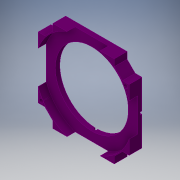
# Autodesk Inventor part: 20_Cube_Insert_CirAp_Lid
Saved by Autodesk Inventor 2019.4 (Build 234330000, 330)
## iProperties
Created: 2019-10-23
Part Number: 20_Cube_Insert_CirAp_Lid
Material: Generic
Document SubType Name: Modeling
Designer: marsikovabarbora
Density: 1 g/cm^3
Appearance: Default
Author: marsikovabarbora
Autodesk Inventor part; units mm, degrees
ref_plane "YZ Plane" through (0, 0, 0) normal (1, 0, 0) x (0, 1, 0)
ref_plane "XZ Plane" through (0, 0, 0) normal (0, 1, 0) x (-1, 0, 0)
ref_plane "XY Plane" through (0, 0, 0) normal (0, 0, 1) x (1, 0, 0)
sketch "Sketch1" plane through (0, 0, 0) normal (0, 0, 1) x (1, 0, 0)
  line L0 (-34.8609, 0) -> (34.8609, 0) construction
  line L1 (0, -34.8609) -> (0, 34.8609) construction
  line L2 (0, 0) -> (11.6542, 11.6542) construction
  line L3 (0, 0) -> (16.4815, 0) construction
  line L4 (0, 24.9006) -> (16.8, 24.9006)
  line L5 (16.8, 24.9006) -> (16.8, 21.2406)
  line L6 (16.8, 21.2406) -> (19.0203, 19.0203)
  line L7 (24.9006, 0) -> (24.9006, 16.8)
  line L8 (24.9006, 16.8) -> (21.2406, 16.8)
  line L9 (21.2406, 16.8) -> (19.0203, 19.0203)
  line L10 (0, 0) -> (-11.6542, 11.6542) construction
  line L11 (0, 0) -> (-16.4815, 0) construction
  line L12 (0, 24.9006) -> (-16.8, 24.9006)
  line L13 (-16.8, 24.9006) -> (-16.8, 21.2406)
  line L14 (-16.8, 21.2406) -> (-19.0203, 19.0203)
  line L15 (-24.9006, 0) -> (-24.9006, 16.8)
  line L16 (-24.9006, 16.8) -> (-21.2406, 16.8)
  line L17 (-21.2406, 16.8) -> (-19.0203, 19.0203)
  line L18 (0, 0) -> (11.6542, -11.6542) construction
  line L19 (0, -24.9006) -> (16.8, -24.9006)
  line L20 (16.8, -24.9006) -> (16.8, -21.2406)
  line L21 (16.8, -21.2406) -> (19.0203, -19.0203)
  line L22 (24.9006, 0) -> (24.9006, -16.8)
  line L23 (24.9006, -16.8) -> (21.2406, -16.8)
  line L24 (21.2406, -16.8) -> (19.0203, -19.0203)
  line L25 (0, 0) -> (-11.6542, -11.6542) construction
  line L26 (0, -24.9006) -> (-16.8, -24.9006)
  line L27 (-16.8, -24.9006) -> (-16.8, -21.2406)
  line L28 (-16.8, -21.2406) -> (-19.0203, -19.0203)
  line L29 (-24.9006, 0) -> (-24.9006, -16.8)
  line L30 (-24.9006, -16.8) -> (-21.2406, -16.8)
  line L31 (-21.2406, -16.8) -> (-19.0203, -19.0203)
  dimension "d0" = 45
  dimension "d1" = 3.14
  dimension "d2" = 3.66
  dimension "d3" = 16.8
  constraints: 60 end point, 24 symmetric about line, 5 point on line, 2 horizontal, 2 perpendicular, 1 equal length
  measures "d0" angle of L3 L2
  measures "d1" distance of L5.end L6.end
  measures "d2" distance of L4.end L5.end
  measures "d3" distance of L4.start L4.end
extrude "Extrusion1" add sketch "Sketch1" along normal blind 2.5
hole "Hole1" at (0, 0, 0) direction (0, 0, 1) diameter 40 end through all
sketch "Sketch5" plane through (0, 0, 2.5) normal (0, 0, 1) x (1, 0, 0)
  circle A0 centre (-22.1796, -5.0624) radius 1.25 construction
  circle A1 centre (-17.7867, 14.1844) radius 1.25 construction
  circle A2 centre (0, 22.75) radius 1.25 construction
  arc A3 (5.9445, 23.5204) -> (2.0147, 24.1761) centre (3.9503, 23.6727) ccw construction
  line L0 (2.0147, 24.1761) -> (2, 24) construction
  arc A4 (2, 24) -> (1.9973, 24.1039) centre (0, 24) ccw construction
  arc A5 (1.9973, 24.1039) -> (1.9775, 24.0019) centre (3.9503, 23.6727) ccw construction
  line L1 (1.9775, 24.0019) -> (1.9921, 24.178) construction
  arc A6 (1.9921, 24.178) -> (-1.9921, 24.178) centre (0, 24) ccw construction
  line L2 (-1.9921, 24.178) -> (-1.9775, 24.0019) construction
  arc A7 (-1.9775, 24.0019) -> (-1.9973, 24.1039) centre (-3.9503, 23.6727) ccw construction
  arc A8 (-1.9973, 24.1039) -> (-2, 24) centre (0, 24) ccw construction
  line L3 (-2, 24) -> (-2.0147, 24.1761) construction
  arc A9 (-2.0147, 24.1761) -> (-5.9445, 23.5204) centre (-3.9503, 23.6727) ccw construction
  line L4 (-5.9445, 23.5204) -> (-5.9012, 23.349) construction
  arc A10 (-5.9012, 23.349) -> (-5.9374, 23.4464) centre (-7.7928, 22.6996) ccw construction
  arc A11 (-5.9374, 23.4464) -> (-5.923, 23.3435) centre (-3.9503, 23.6727) ccw construction
  line L5 (-5.923, 23.3435) -> (-5.9665, 23.5148) construction
  arc A12 (-5.9665, 23.5148) -> (-9.7347, 22.2212) centre (-7.7928, 22.6996) ccw construction
  line L6 (-9.7347, 22.2212) -> (-9.6638, 22.0593) construction
  arc A13 (-9.6638, 22.0593) -> (-9.7156, 22.1493) centre (-11.4227, 21.1074) ccw construction
  arc A14 (-9.7156, 22.1493) -> (-9.6844, 22.0502) centre (-7.7928, 22.6996) ccw construction
  line L7 (-9.6844, 22.0502) -> (-9.7555, 22.212) construction
  arc A15 (-9.7555, 22.212) -> (-13.2594, 20.3158) centre (-11.4227, 21.1074) ccw construction
  line L8 (-13.2594, 20.3158) -> (-13.1628, 20.1678) construction
  arc A16 (-13.1628, 20.1678) -> (-13.2287, 20.2481) centre (-14.7411, 18.9394) ccw construction
  arc A17 (-13.2287, 20.2481) -> (-13.1817, 20.1555) centre (-11.4227, 21.1074) ccw construction
  line L9 (-13.1817, 20.1555) -> (-13.2784, 20.3034) construction
  arc A18 (-13.2784, 20.3034) -> (-16.4225, 17.8563) centre (-14.7411, 18.9394) ccw construction
  line L10 (-16.4225, 17.8563) -> (-16.3028, 17.7262) construction
  arc A19 (-16.3028, 17.7262) -> (-16.381, 17.7946) centre (-17.6574, 16.2548) ccw construction
  arc A20 (-16.381, 17.7946) -> (-16.3194, 17.7109) centre (-14.7411, 18.9394) ccw construction
  line L11 (-16.3194, 17.7109) -> (-16.4392, 17.8409) construction
  arc A21 (-16.4392, 17.8409) -> (-19.1375, 14.9097) centre (-17.6574, 16.2548) ccw construction
  line L12 (-19.1375, 14.9097) -> (-18.9981, 14.8011) construction
  arc A22 (-18.9981, 14.8011) -> (-19.0865, 14.8556) centre (-20.092, 13.1268) ccw construction
  arc A23 (-19.0865, 14.8556) -> (-19.0119, 14.7833) centre (-17.6574, 16.2548) ccw construction
  line L13 (-19.0119, 14.7833) -> (-19.1515, 14.8918) construction
  arc A24 (-19.1515, 14.8918) -> (-21.3306, 11.5564) centre (-20.092, 13.1268) ccw construction
  line L14 (-21.3306, 11.5564) -> (-21.1752, 11.4722) construction
  arc A25 (-21.1752, 11.4722) -> (-21.2714, 11.5115) centre (-21.9786, 9.6407) ccw construction
  arc A26 (-21.2714, 11.5115) -> (-21.1859, 11.4524) centre (-20.092, 13.1268) ccw construction
  line L15 (-21.1859, 11.4524) -> (-21.3414, 11.5365) construction
  arc A27 (-21.3414, 11.5365) -> (-22.9418, 7.8879) centre (-21.9786, 9.6407) ccw construction
  line L16 (-22.9418, 7.8879) -> (-22.7746, 7.8305) construction
  arc A28 (-22.7746, 7.8305) -> (-22.876, 7.8533) centre (-23.2656, 5.8917) ccw construction
  arc A29 (-22.876, 7.8533) -> (-22.782, 7.8091) centre (-21.9786, 9.6407) ccw construction
  line L17 (-22.782, 7.8091) -> (-22.9492, 7.8665) construction
  arc A30 (-22.9492, 7.8665) -> (-23.9272, 4.0042) centre (-23.2656, 5.8917) ccw construction
  line L18 (-23.9272, 4.0042) -> (-23.7529, 3.9751) construction
  arc A31 (-23.7529, 3.9751) -> (-23.8566, 3.981) centre (-23.918, 1.9819) ccw construction
  arc A32 (-23.8566, 3.981) -> (-23.7566, 3.9529) centre (-23.2656, 5.8917) ccw construction
  line L19 (-23.7566, 3.9529) -> (-23.9309, 3.9819) construction
  arc A33 (-23.9309, 3.9819) -> (-24.2599, 0.0113) centre (-23.918, 1.9819) ccw construction
  line L20 (-24.2599, 0.0113) -> (-24.0832, 0.0113) construction
  arc A34 (-24.0832, 0.0113) -> (-24.1865, 0) centre (-23.918, -1.9819) ccw construction
  arc A35 (-24.1865, 0) -> (-24.0832, -0.0113) centre (-23.918, 1.9819) ccw construction
  line L21 (-24.0832, -0.0113) -> (-24.2599, -0.0113) construction
  arc A36 (-24.2599, -0.0113) -> (-23.9309, -3.9819) centre (-23.918, -1.9819) ccw construction
  line L22 (-23.9309, -3.9819) -> (-23.7566, -3.9529) construction
  arc A37 (-23.7566, -3.9529) -> (-23.8566, -3.981) centre (-23.2656, -5.8917) ccw construction
  arc A38 (-23.8566, -3.981) -> (-23.7529, -3.9751) centre (-23.918, -1.9819) ccw construction
  line L23 (-23.7529, -3.9751) -> (-23.9272, -4.0042) construction
  arc A39 (-23.9272, -4.0042) -> (-22.9492, -7.8665) centre (-23.2656, -5.8917) ccw construction
  line L24 (-22.9492, -7.8665) -> (-22.782, -7.8091) construction
  arc A40 (-22.782, -7.8091) -> (-22.876, -7.8533) centre (-21.9786, -9.6407) ccw construction
  arc A41 (-22.876, -7.8533) -> (-22.7746, -7.8305) centre (-23.2656, -5.8917) ccw construction
  line L25 (-22.7746, -7.8305) -> (-22.9418, -7.8879) construction
  arc A42 (-22.9418, -7.8879) -> (-21.3414, -11.5365) centre (-21.9786, -9.6407) ccw construction
  line L26 (-21.3414, -11.5365) -> (-21.1859, -11.4524) construction
  arc A43 (-21.1859, -11.4524) -> (-21.2714, -11.5115) centre (-20.092, -13.1268) ccw construction
  arc A44 (-21.2714, -11.5115) -> (-21.1752, -11.4722) centre (-21.9786, -9.6407) ccw construction
  line L27 (-21.1752, -11.4722) -> (-21.3306, -11.5564) construction
  arc A45 (-21.3306, -11.5564) -> (-19.1515, -14.8918) centre (-20.092, -13.1268) ccw construction
  line L28 (-19.1515, -14.8918) -> (-19.0119, -14.7833) construction
  arc A46 (-19.0119, -14.7833) -> (-19.0865, -14.8556) centre (-17.6574, -16.2548) ccw construction
  arc A47 (-19.0865, -14.8556) -> (-18.9981, -14.8011) centre (-20.092, -13.1268) ccw construction
  line L29 (-18.9981, -14.8011) -> (-19.1375, -14.9097) construction
  arc A48 (-19.1375, -14.9097) -> (-16.4392, -17.8409) centre (-17.6574, -16.2548) ccw construction
  line L30 (-16.4392, -17.8409) -> (-16.3194, -17.7109) construction
  arc A49 (-16.3194, -17.7109) -> (-16.381, -17.7946) centre (-14.7411, -18.9394) ccw construction
  arc A50 (-16.381, -17.7946) -> (-16.3028, -17.7262) centre (-17.6574, -16.2548) ccw construction
  line L31 (-16.3028, -17.7262) -> (-16.4225, -17.8563) construction
  arc A51 (-16.4225, -17.8563) -> (-13.2784, -20.3034) centre (-14.7411, -18.9394) ccw construction
  line L32 (-13.2784, -20.3034) -> (-13.1817, -20.1555) construction
  arc A52 (-13.1817, -20.1555) -> (-13.2287, -20.2481) centre (-11.4227, -21.1074) ccw construction
  arc A53 (-13.2287, -20.2481) -> (-13.1628, -20.1678) centre (-14.7411, -18.9394) ccw construction
  line L33 (-13.1628, -20.1678) -> (-13.2594, -20.3158) construction
  arc A54 (-13.2594, -20.3158) -> (-9.7555, -22.212) centre (-11.4227, -21.1074) ccw construction
  line L34 (-9.7555, -22.212) -> (-9.6844, -22.0502) construction
  arc A55 (-9.6844, -22.0502) -> (-9.7156, -22.1493) centre (-7.7928, -22.6996) ccw construction
  arc A56 (-9.7156, -22.1493) -> (-9.6638, -22.0593) centre (-11.4227, -21.1074) ccw construction
  line L35 (-9.6638, -22.0593) -> (-9.7347, -22.2212) construction
  arc A57 (-9.7347, -22.2212) -> (-5.9665, -23.5148) centre (-7.7928, -22.6996) ccw construction
  line L36 (-5.9665, -23.5148) -> (-5.923, -23.3435) construction
  arc A58 (-5.923, -23.3435) -> (-5.9374, -23.4464) centre (-3.9503, -23.6727) ccw construction
  arc A59 (-5.9374, -23.4464) -> (-5.9012, -23.349) centre (-7.7928, -22.6996) ccw construction
  line L37 (-5.9012, -23.349) -> (-5.9445, -23.5204) construction
  arc A60 (-5.9445, -23.5204) -> (-2.0147, -24.1761) centre (-3.9503, -23.6727) ccw construction
  line L38 (-2.0147, -24.1761) -> (-2, -24) construction
  arc A61 (-2, -24) -> (-1.9973, -24.1039) centre (0, -24) ccw construction
  arc A62 (-1.9973, -24.1039) -> (-1.9775, -24.0019) centre (-3.9503, -23.6727) ccw construction
  line L39 (-1.9775, -24.0019) -> (-1.9921, -24.178) construction
  arc A63 (-1.9921, -24.178) -> (1.9921, -24.178) centre (0, -24) ccw construction
  line L40 (1.9921, -24.178) -> (1.9775, -24.0019) construction
  arc A64 (1.9775, -24.0019) -> (1.9973, -24.1039) centre (3.9503, -23.6727) ccw construction
  arc A65 (1.9973, -24.1039) -> (2, -24) centre (0, -24) ccw construction
  line L41 (2, -24) -> (2.0147, -24.1761) construction
  arc A66 (2.0147, -24.1761) -> (5.9445, -23.5204) centre (3.9503, -23.6727) ccw construction
  line L42 (5.9445, -23.5204) -> (5.9012, -23.349) construction
  arc A67 (5.9012, -23.349) -> (5.9374, -23.4464) centre (7.7928, -22.6996) ccw construction
  arc A68 (5.9374, -23.4464) -> (5.923, -23.3435) centre (3.9503, -23.6727) ccw construction
  line L43 (5.923, -23.3435) -> (5.9665, -23.5148) construction
  arc A69 (5.9665, -23.5148) -> (9.7347, -22.2212) centre (7.7928, -22.6996) ccw construction
  line L44 (9.7347, -22.2212) -> (9.6638, -22.0593) construction
  arc A70 (9.6638, -22.0593) -> (9.7156, -22.1493) centre (11.4227, -21.1074) ccw construction
  arc A71 (9.7156, -22.1493) -> (9.6844, -22.0502) centre (7.7928, -22.6996) ccw construction
  line L45 (9.6844, -22.0502) -> (9.7555, -22.212) construction
  arc A72 (9.7555, -22.212) -> (13.2594, -20.3158) centre (11.4227, -21.1074) ccw construction
  line L46 (13.2594, -20.3158) -> (13.1628, -20.1678) construction
  arc A73 (13.1628, -20.1678) -> (13.2287, -20.2481) centre (14.7411, -18.9394) ccw construction
  arc A74 (13.2287, -20.2481) -> (13.1817, -20.1555) centre (11.4227, -21.1074) ccw construction
  line L47 (13.1817, -20.1555) -> (13.2784, -20.3034) construction
  arc A75 (13.2784, -20.3034) -> (16.4225, -17.8563) centre (14.7411, -18.9394) ccw construction
  line L48 (16.4225, -17.8563) -> (16.3028, -17.7262) construction
  arc A76 (16.3028, -17.7262) -> (16.381, -17.7946) centre (17.6574, -16.2548) ccw construction
  arc A77 (16.381, -17.7946) -> (16.3194, -17.7109) centre (14.7411, -18.9394) ccw construction
  line L49 (16.3194, -17.7109) -> (16.4392, -17.8409) construction
  arc A78 (16.4392, -17.8409) -> (19.1375, -14.9097) centre (17.6574, -16.2548) ccw construction
  line L50 (19.1375, -14.9097) -> (18.9981, -14.8011) construction
  arc A79 (18.9981, -14.8011) -> (19.0865, -14.8556) centre (20.092, -13.1268) ccw construction
  arc A80 (19.0865, -14.8556) -> (19.0119, -14.7833) centre (17.6574, -16.2548) ccw construction
  line L51 (19.0119, -14.7833) -> (19.1515, -14.8918) construction
  arc A81 (19.1515, -14.8918) -> (21.3306, -11.5564) centre (20.092, -13.1268) ccw construction
  line L52 (21.3306, -11.5564) -> (21.1752, -11.4722) construction
  arc A82 (21.1752, -11.4722) -> (21.2714, -11.5115) centre (21.9786, -9.6407) ccw construction
  arc A83 (21.2714, -11.5115) -> (21.1859, -11.4524) centre (20.092, -13.1268) ccw construction
  line L53 (21.1859, -11.4524) -> (21.3414, -11.5365) construction
  arc A84 (21.3414, -11.5365) -> (22.9418, -7.8879) centre (21.9786, -9.6407) ccw construction
  line L54 (22.9418, -7.8879) -> (22.7746, -7.8305) construction
  arc A85 (22.7746, -7.8305) -> (22.876, -7.8533) centre (23.2656, -5.8917) ccw construction
  arc A86 (22.876, -7.8533) -> (22.782, -7.8091) centre (21.9786, -9.6407) ccw construction
  line L55 (22.782, -7.8091) -> (22.9492, -7.8665) construction
  arc A87 (22.9492, -7.8665) -> (23.9272, -4.0042) centre (23.2656, -5.8917) ccw construction
  line L56 (23.9272, -4.0042) -> (23.7529, -3.9751) construction
  arc A88 (23.7529, -3.9751) -> (23.8566, -3.981) centre (23.918, -1.9819) ccw construction
  arc A89 (23.8566, -3.981) -> (23.7566, -3.9529) centre (23.2656, -5.8917) ccw construction
  line L57 (23.7566, -3.9529) -> (23.9309, -3.9819) construction
  arc A90 (23.9309, -3.9819) -> (24.2599, -0.0113) centre (23.918, -1.9819) ccw construction
  line L58 (24.2599, -0.0113) -> (24.0832, -0.0113) construction
  arc A91 (24.0832, -0.0113) -> (24.1865, 0) centre (23.918, 1.9819) ccw construction
  arc A92 (24.1865, 0) -> (24.0832, 0.0113) centre (23.918, -1.9819) ccw construction
  line L59 (24.0832, 0.0113) -> (24.2599, 0.0113) construction
  arc A93 (24.2599, 0.0113) -> (23.9309, 3.9819) centre (23.918, 1.9819) ccw construction
  line L60 (23.9309, 3.9819) -> (23.7566, 3.9529) construction
  arc A94 (23.7566, 3.9529) -> (23.8566, 3.981) centre (23.2656, 5.8917) ccw construction
  arc A95 (23.8566, 3.981) -> (23.7529, 3.9751) centre (23.918, 1.9819) ccw construction
  line L61 (23.7529, 3.9751) -> (23.9272, 4.0042) construction
  arc A96 (23.9272, 4.0042) -> (22.9492, 7.8665) centre (23.2656, 5.8917) ccw construction
  line L62 (22.9492, 7.8665) -> (22.782, 7.8091) construction
  arc A97 (22.782, 7.8091) -> (22.876, 7.8533) centre (21.9786, 9.6407) ccw construction
  arc A98 (22.876, 7.8533) -> (22.7746, 7.8305) centre (23.2656, 5.8917) ccw construction
  line L63 (22.7746, 7.8305) -> (22.9418, 7.8879) construction
  arc A99 (22.9418, 7.8879) -> (21.3414, 11.5365) centre (21.9786, 9.6407) ccw construction
  line L64 (21.3414, 11.5365) -> (21.1859, 11.4524) construction
  arc A100 (21.1859, 11.4524) -> (21.2714, 11.5115) centre (20.092, 13.1268) ccw construction
  arc A101 (21.2714, 11.5115) -> (21.1752, 11.4722) centre (21.9786, 9.6407) ccw construction
  line L65 (21.1752, 11.4722) -> (21.3306, 11.5564) construction
  arc A102 (21.3306, 11.5564) -> (19.1515, 14.8918) centre (20.092, 13.1268) ccw construction
  line L66 (19.1515, 14.8918) -> (19.0119, 14.7833) construction
  arc A103 (19.0119, 14.7833) -> (19.0865, 14.8556) centre (17.6574, 16.2548) ccw construction
  arc A104 (19.0865, 14.8556) -> (18.9981, 14.8011) centre (20.092, 13.1268) ccw construction
  line L67 (18.9981, 14.8011) -> (19.1375, 14.9097) construction
  arc A105 (19.1375, 14.9097) -> (16.4392, 17.8409) centre (17.6574, 16.2548) ccw construction
  line L68 (16.4392, 17.8409) -> (16.3194, 17.7109) construction
  arc A106 (16.3194, 17.7109) -> (16.381, 17.7946) centre (14.7411, 18.9394) ccw construction
  arc A107 (16.381, 17.7946) -> (16.3028, 17.7262) centre (17.6574, 16.2548) ccw construction
  line L69 (16.3028, 17.7262) -> (16.4225, 17.8563) construction
  arc A108 (16.4225, 17.8563) -> (13.2784, 20.3034) centre (14.7411, 18.9394) ccw construction
  line L70 (13.2784, 20.3034) -> (13.1817, 20.1555) construction
  arc A109 (13.1817, 20.1555) -> (13.2287, 20.2481) centre (11.4227, 21.1074) ccw construction
  arc A110 (13.2287, 20.2481) -> (13.1628, 20.1678) centre (14.7411, 18.9394) ccw construction
  line L71 (13.1628, 20.1678) -> (13.2594, 20.3158) construction
  arc A111 (13.2594, 20.3158) -> (9.7555, 22.212) centre (11.4227, 21.1074) ccw construction
  line L72 (9.7555, 22.212) -> (9.6844, 22.0502) construction
  arc A112 (9.6844, 22.0502) -> (9.7156, 22.1493) centre (7.7928, 22.6996) ccw construction
  arc A113 (9.7156, 22.1493) -> (9.6638, 22.0593) centre (11.4227, 21.1074) ccw construction
  line L73 (9.6638, 22.0593) -> (9.7347, 22.2212) construction
  arc A114 (9.7347, 22.2212) -> (5.9665, 23.5148) centre (7.7928, 22.6996) ccw construction
  line L74 (5.9665, 23.5148) -> (5.923, 23.3435) construction
  arc A115 (5.923, 23.3435) -> (5.9374, 23.4464) centre (3.9503, 23.6727) ccw construction
  arc A116 (5.9374, 23.4464) -> (5.9012, 23.349) centre (7.7928, 22.6996) ccw construction
  line L75 (5.9012, 23.349) -> (5.9445, 23.5204) construction
  circle A117 centre (0, 0) radius 21 construction
  circle A118 centre (0, 0) radius 20 construction
  line L76 (16.8, 24.9006) -> (-16.8, 24.9006) construction
  line L77 (-16.8, 24.9006) -> (-16.8, 21.2406) construction
  line L78 (-16.8, 21.2406) -> (-21.2406, 16.8) construction
  line L79 (-21.2406, 16.8) -> (-24.9006, 16.8) construction
  line L80 (-24.9006, 16.8) -> (-24.9006, -16.8) construction
  line L81 (-24.9006, -16.8) -> (-21.2406, -16.8) construction
  line L82 (-21.2406, -16.8) -> (-16.8, -21.2406) construction
  line L83 (-16.8, -21.2406) -> (-16.8, -24.9006) construction
  line L84 (-16.8, -24.9006) -> (16.8, -24.9006) construction
  line L85 (16.8, -24.9006) -> (16.8, -21.2406) construction
  line L86 (16.8, -21.2406) -> (21.2406, -16.8) construction
  line L87 (21.2406, -16.8) -> (24.9006, -16.8) construction
  line L88 (24.9006, -16.8) -> (24.9006, 16.8) construction
  line L89 (24.9006, 16.8) -> (21.2406, 16.8) construction
  line L90 (21.2406, 16.8) -> (16.8, 21.2406) construction
  line L91 (16.8, 21.2406) -> (16.8, 24.9006) construction
  circle A119 centre (0, 0) radius 26 construction
  line L92 (-16.8, 24.9006) -> (16.8, 24.9006) projected
  line L93 (-9.0669, 24.9006) -> (-16.8, 24.9006)
  line L94 (-16.8, 24.9006) -> (-16.8, 21.2406)
  line L95 (-16.8, 21.2406) -> (-21.2406, 16.8)
  line L96 (-24.9006, 16.8) -> (-21.2406, 16.8) projected
  line L97 (-21.2406, 16.8) -> (-24.9006, 16.8)
  line L98 (-24.9006, 16.8) -> (-24.9006, 9.0669)
  line L99 (-24.9006, 16.8) -> (-24.9006, -16.8) projected
  arc A120 (-9.0669, 24.9006) -> (-24.9006, 9.0669) centre (0, 0) ccw
  circle A121 centre (17.7867, 14.1844) radius 1.25 projected
  circle A122 centre (22.1796, -5.0624) radius 1.25 projected
  circle A123 centre (9.8709, -20.497) radius 1.25 projected
  circle A124 centre (-9.8709, -20.497) radius 1.25 projected
  dimension "d20" = 0.5
  constraints: 10 end point, 3 collinear, 2 centre point, 2 point on circle, 2 point on line, 1 coincident, 1 tangent
  measures "d20" radial gap between concentric circles of A120 A119
extrude "Extrusion3" add sketch "Sketch5" along normal blind 4.5 contours L92 A120 L98 L96 L95 L94
pattern_circular "Circular Pattern1" count 4 over 360 about axis through (0, 0, -10) along (0, 0, 1) of "Extrusion3"
sketch "Sketch6" plane through (9.0669, 24.9006, 7) normal (0, 0, 1) x (1, 0, 0)
  line L0 (15.8337, -8.1006) -> (12.1737, -8.1006) construction
  line L1 (12.1737, -8.1006) -> (7.7331, -3.66) construction
  line L2 (7.7331, -3.66) -> (7.7331, 0) construction
  line L3 (7.7331, 0) -> (0, 0) construction
  arc A0 (15.8337, -15.8337) -> (0, 0) centre (-9.0669, -24.9006) ccw construction
  line L4 (15.8337, -15.8337) -> (15.8337, -8.1006) construction
  line L5 (-33.9675, -41.7006) -> (-30.3075, -41.7006) construction
  line L6 (-30.3075, -41.7006) -> (-25.8669, -46.1413) construction
  line L7 (-25.8669, -46.1413) -> (-25.8669, -49.8013) construction
  line L8 (-25.8669, -49.8013) -> (-18.1338, -49.8013) construction
  arc A1 (-33.9675, -33.9675) -> (-18.1338, -49.8013) centre (-9.0669, -24.9006) ccw construction
  line L9 (-33.9675, -33.9675) -> (-33.9675, -41.7006) construction
  circle A2 centre (-32.1675, -39.9006) radius 1.05
  circle A3 centre (14.0337, -9.9006) radius 1.05
  line L10 (-33.9675, -41.7006) -> (-32.1675, -41.7006) construction
  line L11 (-32.1675, -41.7006) -> (-32.1675, -39.9006) construction
  line L12 (-32.1675, -39.9006) -> (-33.9675, -39.9006) construction
  line L13 (-33.9675, -39.9006) -> (-33.9675, -41.7006) construction
  line L14 (7.7331, 0) -> (6.2331, 0) construction
  line L15 (7.7331, -1.5) -> (7.7331, 0) construction
  line L16 (12.1737, -8.1006) -> (15.8337, -8.1006) projected
  line L17 (14.0337, -8.1006) -> (14.0337, -9.9006) construction
  line L18 (14.0337, -9.9006) -> (15.8337, -9.9006) construction
  line L19 (15.8337, -8.1006) -> (15.8337, -41.7006) projected
  dimension "d26" = 2.1
  dimension "d27" = 2.1
  dimension "d28" = 1.8
  dimension "d29" = 1.8
  dimension "d34" = 1.8
  dimension "d35" = 1.8
  constraints: 16 end point, 3 perpendicular, 2 centre point, 2 horizontal, 2 parallel, 2 point on line, 1 coincident
  measures "d26" diameter of A2
  measures "d27" diameter of A3
  measures "d28" distance of L11.end L12.end
  measures "d29" distance of L10.end L11.end
  measures "d34" distance from line of L4 A3.centre
  measures "d35" distance from line of L0 A3.centre
extrude "Extrusion4" cut sketch "Sketch6" against normal through all
sketch "Skizze7" plane through (0, 0, 0) normal (0, 0, -1) x (-1, 0, 0)
  line L0 (-2.425, 24.184) -> (2.4258, 24.184) construction
  line L1 (2.4258, 24.184) -> (2.4258, 22.0206) construction
  line L2 (2.4258, 22.0206) -> (-2.425, 22.0206) construction
  line L3 (-2.425, 22.0206) -> (-2.425, 24.184) construction
  line L4 (20.3128, 1.6063) -> (24.5736, 1.6063) construction
  line L5 (24.5736, 1.6063) -> (24.5736, -1.3314) construction
  line L6 (24.5736, -1.3314) -> (20.3128, -1.3314) construction
  line L7 (20.3128, -1.3314) -> (20.3128, 1.6063) construction
  line L8 (-24.9006, 16.8) -> (-24.9006, -16.8) projected
  circle A0 centre (0, 0) radius 20 projected
  line L9 (-16.8, -24.9006) -> (16.8, -24.9006) projected
  spline S0 degree 2 poles (-2.2867, 23.1317) (-2.2867, 23.3664) (-2.1336, 23.7567) (-2.0002, 23.8974) knots 0 0 0 1 2 2 2
  spline S1 degree 2 poles (-2.0002, 23.8974) (-1.8742, 24.0333) (-1.5062, 24.184) (-1.3185, 24.184) knots 0 0 0 1 2 2 2
  spline S2 degree 2 poles (-1.3185, 24.184) (-1.1085, 24.184) (-0.7677, 24.0432) (-0.6417, 23.9098) knots 0 0 0 1 2 2 2
  spline S3 degree 2 poles (-0.6417, 23.9098) (-0.4836, 23.7418) (-0.3107, 23.1984) (-0.3107, 22.781) knots 0 0 0 1 2 2 2
  spline S4 degree 2 poles (-0.3107, 22.781) (-0.3107, 22.4031) (-0.4811, 21.7263) (-0.6466, 21.5015) knots 0 0 0 1 2 2 2
  spline S5 degree 2 poles (-0.6466, 21.5015) (-0.822, 21.2644) (-1.316, 21.0149) (-1.6766, 21.0149) knots 0 0 0 1 2 2 2
  spline S6 degree 2 poles (-1.6766, 21.0149) (-1.7581, 21.0149) (-1.9434, 21.0322) (-2.0224, 21.0569) knots 0 0 0 1 2 2 2
  line L10 (-2.0224, 21.0569) -> (-2.0224, 21.4497)
  line L11 (-2.0224, 21.4497) -> (-2.0027, 21.4497)
  spline S7 degree 2 poles (-2.0027, 21.4497) (-1.9508, 21.42) (-1.7334, 21.3681) (-1.6223, 21.3681) knots 0 0 0 1 2 2 2
  spline S8 degree 2 poles (-1.6223, 21.3681) (-1.2221, 21.3681) (-0.7652, 21.8967) (-0.7331, 22.3858) knots 0 0 0 1 2 2 2
  spline S9 degree 2 poles (-0.7331, 22.3858) (-0.8961, 22.2746) (-1.1925, 22.1734) (-1.3679, 22.1734) knots 0 0 0 1 2 2 2
  spline S10 degree 2 poles (-1.3679, 22.1734) (-1.5358, 22.1734) (-1.8149, 22.2475) (-1.9557, 22.3537) knots 0 0 0 1 2 2 2
  spline S11 degree 2 poles (-1.9557, 22.3537) (-2.1188, 22.4797) (-2.2867, 22.8625) (-2.2867, 23.1317) knots 0 0 0 1 2 2 2
  spline S12 degree 2 poles (-0.7232, 22.8724) (-0.7232, 23.1811) (-0.8368, 23.5714) (-0.9381, 23.6776) knots 0 0 0 1 2 2 2
  spline S13 degree 2 poles (-0.9381, 23.6776) (-1.027, 23.7764) (-1.2123, 23.8505) (-1.3209, 23.8505) knots 0 0 0 1 2 2 2
  spline S14 degree 2 poles (-1.3209, 23.8505) (-1.5729, 23.8505) (-1.8718, 23.4899) (-1.8718, 23.149) knots 0 0 0 1 2 2 2
  spline S15 degree 2 poles (-1.8718, 23.149) (-1.8718, 22.9564) (-1.773, 22.7069) (-1.6643, 22.618) knots 0 0 0 1 2 2 2
  spline S16 degree 2 poles (-1.6643, 22.618) (-1.5852, 22.5538) (-1.3901, 22.5118) (-1.2765, 22.5118) knots 0 0 0 1 2 2 2
  spline S17 degree 2 poles (-1.2765, 22.5118) (-1.1456, 22.5118) (-0.8442, 22.6032) (-0.7306, 22.6797) knots 0 0 0 1 2 2 2
  spline S18 degree 2 poles (-0.7306, 22.6797) (-0.7281, 22.7094) (-0.7232, 22.8106) (-0.7232, 22.8724) knots 0 0 0 1 2 2 2
  spline S19 degree 2 poles (1.9815, 22.5982) (1.9815, 21.7782) (1.5048, 21.01) (1.0083, 21.01) knots 0 0 0 1 2 2 2
  spline S20 degree 2 poles (1.0083, 21.01) (0.5044, 21.01) (0.0326, 21.793) (0.0326, 22.5957) knots 0 0 0 1 2 2 2
  spline S21 degree 2 poles (0.0326, 22.5957) (0.0326, 23.4207) (0.5093, 24.184) (1.0083, 24.184) knots 0 0 0 1 2 2 2
  spline S22 degree 2 poles (1.0083, 24.184) (1.5097, 24.184) (1.9815, 23.3936) (1.9815, 22.5982) knots 0 0 0 1 2 2 2
  spline S23 degree 2 poles (1.4578, 21.6695) (1.5171, 21.8202) (1.5665, 22.2845) (1.5665, 22.5982) knots 0 0 0 1 2 2 2
  spline S24 degree 2 poles (1.5665, 22.5982) (1.5665, 22.9119) (1.5171, 23.3738) (1.4554, 23.5294) knots 0 0 0 1 2 2 2
  spline S25 degree 2 poles (1.4554, 23.5294) (1.3936, 23.685) (1.1787, 23.8456) (1.0083, 23.8456) knots 0 0 0 1 2 2 2
  spline S26 degree 2 poles (1.0083, 23.8456) (0.8379, 23.8456) (0.618, 23.685) (0.5538, 23.5245) knots 0 0 0 1 2 2 2
  spline S27 degree 2 poles (0.5538, 23.5245) (0.4921, 23.3689) (0.4476, 22.8946) (0.4476, 22.5957) knots 0 0 0 1 2 2 2
  spline S28 degree 2 poles (0.4476, 22.5957) (0.4476, 22.2746) (0.4871, 21.8449) (0.5513, 21.6769) knots 0 0 0 1 2 2 2
  spline S29 degree 2 poles (0.5513, 21.6769) (0.6106, 21.5188) (0.8304, 21.3484) (1.0083, 21.3484) knots 0 0 0 1 2 2 2
  spline S30 degree 2 poles (1.0083, 21.3484) (1.1762, 21.3484) (1.3961, 21.5089) (1.4578, 21.6695) knots 0 0 0 1 2 2 2
  spline S31 degree 2 poles (3.9155, 23.396) (3.9155, 23.0675) (3.466, 22.618) (3.1374, 22.618) knots 0 0 0 1 2 2 2
  spline S32 degree 2 poles (3.1374, 22.618) (2.8114, 22.618) (2.3569, 23.065) (2.3569, 23.396) knots 0 0 0 1 2 2 2
  spline S33 degree 2 poles (2.3569, 23.396) (2.3569, 23.7245) (2.8065, 24.1741) (3.1374, 24.1741) knots 0 0 0 1 2 2 2
  spline S34 degree 2 poles (3.1374, 24.1741) (3.466, 24.1741) (3.9155, 23.7245) (3.9155, 23.396) knots 0 0 0 1 2 2 2
  spline S35 degree 2 poles (3.5944, 23.396) (3.5944, 23.5936) (3.3326, 23.8629) (3.1374, 23.8629) knots 0 0 0 1 2 2 2
  spline S36 degree 2 poles (3.1374, 23.8629) (2.9398, 23.8629) (2.678, 23.5936) (2.678, 23.396) knots 0 0 0 1 2 2 2
  spline S37 degree 2 poles (2.678, 23.396) (2.678, 23.196) (2.9448, 22.9292) (3.1374, 22.9292) knots 0 0 0 1 2 2 2
  spline S38 degree 2 poles (3.1374, 22.9292) (3.3326, 22.9292) (3.5944, 23.2009) (3.5944, 23.396) knots 0 0 0 1 2 2 2
  spline S39 degree 2 poles (22.4321, 0.0205) (22.4321, -0.7995) (21.9554, -1.5677) (21.4589, -1.5677) knots 0 0 0 1 2 2 2
  spline S40 degree 2 poles (21.4589, -1.5677) (20.955, -1.5677) (20.4832, -0.7847) (20.4832, 0.0181) knots 0 0 0 1 2 2 2
  spline S41 degree 2 poles (20.4832, 0.0181) (20.4832, 0.8431) (20.9599, 1.6063) (21.4589, 1.6063) knots 0 0 0 1 2 2 2
  spline S42 degree 2 poles (21.4589, 1.6063) (21.9603, 1.6063) (22.4321, 0.8159) (22.4321, 0.0205) knots 0 0 0 1 2 2 2
  spline S43 degree 2 poles (21.9084, -0.9082) (21.9677, -0.7575) (22.0171, -0.2932) (22.0171, 0.0205) knots 0 0 0 1 2 2 2
  spline S44 degree 2 poles (22.0171, 0.0205) (22.0171, 0.3342) (21.9677, 0.7961) (21.906, 0.9517) knots 0 0 0 1 2 2 2
  spline S45 degree 2 poles (21.906, 0.9517) (21.8442, 1.1073) (21.6293, 1.2679) (21.4589, 1.2679) knots 0 0 0 1 2 2 2
  spline S46 degree 2 poles (21.4589, 1.2679) (21.2885, 1.2679) (21.0686, 1.1073) (21.0044, 0.9468) knots 0 0 0 1 2 2 2
  spline S47 degree 2 poles (21.0044, 0.9468) (20.9427, 0.7912) (20.8982, 0.3169) (20.8982, 0.0181) knots 0 0 0 1 2 2 2
  spline S48 degree 2 poles (20.8982, 0.0181) (20.8982, -0.303) (20.9377, -0.7328) (21.0019, -0.9008) knots 0 0 0 1 2 2 2
  spline S49 degree 2 poles (21.0019, -0.9008) (21.0612, -1.0589) (21.281, -1.2293) (21.4589, -1.2293) knots 0 0 0 1 2 2 2
  spline S50 degree 2 poles (21.4589, -1.2293) (21.6268, -1.2293) (21.8467, -1.0687) (21.9084, -0.9082) knots 0 0 0 1 2 2 2
  spline S51 degree 2 poles (24.3661, 0.8184) (24.3661, 0.4898) (23.9166, 0.0403) (23.588, 0.0403) knots 0 0 0 1 2 2 2
  spline S52 degree 2 poles (23.588, 0.0403) (23.262, 0.0403) (22.8075, 0.4874) (22.8075, 0.8184) knots 0 0 0 1 2 2 2
  spline S53 degree 2 poles (22.8075, 0.8184) (22.8075, 1.1469) (23.2571, 1.5964) (23.588, 1.5964) knots 0 0 0 1 2 2 2
  spline S54 degree 2 poles (23.588, 1.5964) (23.9166, 1.5964) (24.3661, 1.1469) (24.3661, 0.8184) knots 0 0 0 1 2 2 2
  spline S55 degree 2 poles (24.045, 0.8184) (24.045, 1.016) (23.7832, 1.2852) (23.588, 1.2852) knots 0 0 0 1 2 2 2
  spline S56 degree 2 poles (23.588, 1.2852) (23.3904, 1.2852) (23.1286, 1.016) (23.1286, 0.8184) knots 0 0 0 1 2 2 2
  spline S57 degree 2 poles (23.1286, 0.8184) (23.1286, 0.6183) (23.3954, 0.3515) (23.588, 0.3515) knots 0 0 0 1 2 2 2
  spline S58 degree 2 poles (23.588, 0.3515) (23.7832, 0.3515) (24.045, 0.6232) (24.045, 0.8184) knots 0 0 0 1 2 2 2
  constraints: 4 other
emboss "Prägen1" sketch "Skizze7" operation cut depth 1 direction (0, 0, 1) contours S0 S1 S2 S3 S4 S5 S6 L10 L11 S7 S8 S9 S10 S11 | S19 S20 S21 S22 | S31 S32 S33 S34 | S39 S40 S41 S42 | S51 S52 S53 S54
sketch "Skizze8" plane through (0, 0, 0) normal (0, 0, -1) x (-1, 0, 0)
  line L0 (-24.9006, -9.0669) -> (-24.9006, 9.0669) projected
  line L1 (-24.9006, 0.75) -> (-24.9006, -0.75)
  line L2 (-24.9006, -0.75) -> (-19.9859, -0.75)
  line L3 (9.0669, -24.9006) -> (-9.0669, -24.9006) projected
  line L4 (0.75, -24.9006) -> (-0.75, -24.9006)
  line L5 (-0.75, -24.9006) -> (-0.75, -19.9859)
  arc A0 (-19.9859, 0.75) -> (-19.9859, -0.75) centre (0, 0) ccw
  arc A1 (-0.75, -19.9859) -> (0.75, -19.9859) centre (0, 0) ccw
  line L6 (0.75, -19.9859) -> (0.75, -24.9006)
  line L7 (-19.9859, 0.75) -> (-24.9006, 0.75)
  point P0 (0, 0)
  point P1 (0, -24.9006)
  point P2 (-24.9006, 0)
  point P3 (-24.9006, 0)
  point P4 (-20, 0)
  dimension "d40" = 1.5
  dimension "d41" = 1.5
  constraints: 12 end point, 5 point on circle, 4 point on line, 3 horizontal alignment, 3 midpoint, 2 centre point, 2 parallel, 2 perpendicular, 1 vertical alignment
  measures "d40" distance between parallel lines of L2 L7
  measures "d41" distance between parallel lines of L5 L6
extrude "Extrusion5" cut sketch "Skizze8" against normal blind 1
body "Solid1"
